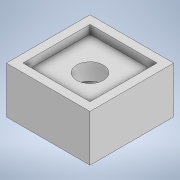
# Autodesk Inventor part: Тестовая модель (деталь в деталь)
Saved by Autodesk Inventor 2020 (Build 240168000, 168)
## iProperties
Created: 2021-04-11
Part Number: Тестовая модель (деталь в деталь)
Material: Типовые
Document SubType Name: Modeling
Designer: Антон
Density: 1 g/cm^3
Appearance: По умолчанию
Author: Антон
Autodesk Inventor part; units mm, degrees
ref_plane "YZ Plane" through (0, 0, 0) normal (1, 0, 0) x (0, 1, 0)
ref_plane "XZ Plane" through (0, 0, 0) normal (0, 1, 0) x (-1, 0, 0)
ref_plane "XY Plane" through (0, 0, 0) normal (0, 0, 1) x (1, 0, 0)
sketch "Эскиз1" plane through (0, 0, 0) normal (0, 1, 0) x (-1, 0, 0)
  line L0 (0, 0) -> (10.05, 0)
  line L1 (10.05, 0) -> (10.05, -10.05)
  line L2 (10.05, -10.05) -> (0, -10.05)
  line L3 (0, -10.05) -> (0, 0)
  dimension "d0" = 10.05
  dimension "d1" = 10.05
  constraints: 8 end point, 2 parallel, 1 horizontal, 1 perpendicular
  measures "d0" distance of L1.end L2.end
  measures "d1" distance of L0.end L1.end
extrude "Выдавливание1" add sketch "Эскиз1" along normal blind 5.6
sketch "Эскиз2" plane through (0, 5.6, 0) normal (0, 1, 0) x (1, 0, 0)
  line L0 (-10.05, 10.05) -> (-10.05, 0) projected
  line L1 (-10.05, 5.025) -> (0, 5.025)
  line L2 (0, 0) -> (0, 10.05) projected
  line L3 (-1, 1) -> (-9.05, 1)
  line L4 (-9.05, 1) -> (-9.05, 9.05)
  line L5 (-9.05, 9.05) -> (-1, 9.05)
  line L6 (-1, 9.05) -> (-1, 1)
  line L7 (-1, 1) -> (-9.05, 9.05) construction
  line L8 (-9.05, 1) -> (-1, 9.05) construction
  point P0 (-5.025, 5.025)
  dimension "d4" = 10.05
  dimension "d5" = 10.05
  dimension "d6" = 8.05
  dimension "d7" = 8.05
  constraints: 14 end point, 5 midpoint, 2 parallel, 1 horizontal, 1 perpendicular
  measures "d4" distance of L0.start L0.end
  measures "d5" distance between parallel lines of L2 L0
  measures "d6" distance of L4.end L5.end
  measures "d7" distance of L3.end L4.end
extrude "Выдавливание2" cut sketch "Эскиз2" against normal blind 1
sketch "Эскиз3" plane through (0, 0, 0) normal (0, -1, 0) x (1, 0, 0)
  line L0 (0, 0) -> (0, -10.05) projected
  line L1 (0, -5.025) -> (-10.05, -5.025)
  line L2 (-10.05, -10.05) -> (-10.05, 0) projected
  point P0 (-5.025, -5.025)
  constraints: 3 midpoint, 2 end point
hole "Отверстие1" at (-5.025, 0, -5.025) direction (0, 1, 0) diameter 3.2 end through all
sketch "Эскиз4" plane through (0, 0, 0) normal (0, -1, 0) x (1, 0, 0)
  circle A0 centre (-5.025, -5.025) radius 1.6 projected
  line L0 (-6.6416, -7.825) -> (-8.2582, -5.025)
  line L1 (-8.2582, -5.025) -> (-6.6416, -2.225)
  line L2 (-6.6416, -2.225) -> (-3.4084, -2.225)
  line L3 (-3.4084, -2.225) -> (-1.7918, -5.025)
  line L4 (-1.7918, -5.025) -> (-3.4084, -7.825)
  line L5 (-3.4084, -7.825) -> (-6.6416, -7.825)
  point P0 (0, 0)
  dimension "d17" = 5.6
  constraints: 12 end point, 1 coincident, 13 other
  measures "d17" distance between parallel lines of L5 L2
extrude "Выдавливание3" cut sketch "Эскиз4" against normal blind 2.6 contours A0 | L0 L1 L2 L3 L4 L5
